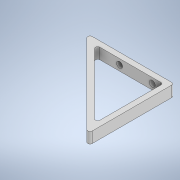
# Autodesk Inventor part: 25degbracketlcd
Saved by Autodesk Inventor 2020.2 (Build 242310000, 310)
## iProperties
Created: 2020-08-26
Part Number: 25degbracketlcd
Material: Generic
Document SubType Name: Modeling
Designer: JK
Density: 1 g/cm^3
Appearance: Default
Author: JK
Autodesk Inventor part; units mm, degrees
ref_plane "YZ Plane" through (0, 0, 0) normal (1, 0, 0) x (0, 1, 0)
ref_plane "XZ Plane" through (0, 0, 0) normal (0, 1, 0) x (-1, 0, 0)
ref_plane "XY Plane" through (0, 0, 0) normal (0, 0, 1) x (1, 0, 0)
sketch "Sketch1" plane through (0, 0, 0) normal (0, 1, 0) x (-1, 0, 0)
  line L0 (62.585, -18.917) -> (-13.8794, 57.5475)
  line L1 (-13.8794, 57.5475) -> (-13.8794, -22.4525)
  line L2 (-13.8794, -22.4525) -> (-8.8794, -22.4525)
  line L3 (-8.8794, -22.4525) -> (-8.8794, 45.4764)
  line L4 (-8.8794, 45.4764) -> (59.0495, -22.4525)
  line L5 (59.0495, -22.4525) -> (62.585, -18.917)
  line L6 (59.0495, -22.4525) -> (-8.8794, -22.4525)
  line L7 (-8.8794, -17.4525) -> (61.1206, -17.4525)
  line L8 (59.0495, -22.4525) -> (66.1206, -22.4525)
  line L9 (66.1206, -22.4525) -> (62.585, -18.917)
  point P0 (0, 0)
  point P1 (54.0495, -17.4525)
  dimension "d0" = 45
  dimension "d1" = 5
  dimension "d3" = 5
  dimension "d7" = 5
  dimension "d27" = 80
  constraints: 20 end point, 2 horizontal, 2 perpendicular, 2 point on line, 2 vertical, 1 collinear, 1 horizontal alignment, 1 parallel
  measures "d0" angle of L4 L3
  measures "d1" distance between parallel lines of L3 L1
  measures "d3" distance between parallel lines of L4 L0
  measures "d7" distance between parallel lines of L6 L7
  measures "d27" distance of L1.end L8.end
extrude "Extrusion1" add sketch "Sketch1" along normal blind 10 contours L5 L4 L7 L0 | L9 L8 L5 | L7 L4 L3 L2 L1 L0 | L6 L3 L7 L4
sketch "Sketch3" plane through (-54.0495, 0, -17.4525) normal (0, 0, 1) x (1, 0, 0)
  circle A0 centre (52.9289, 5) radius 2.75
  line L0 (0, 10) -> (62.9289, 10) projected
  line L1 (67.9289, 0) -> (67.9289, 10) projected
  circle A1 centre (22.9289, 5) radius 2.75
  point P0 (54.0495, 0)
  dimension "d16" = 5.5
  dimension "d17" = 5
  dimension "d18" = 15
  dimension "d22" = 30
  constraints: 2 centre point, 1 equal radius, 1 horizontal alignment
  measures "d16" diameter of A0
  measures "d17" distance from line of L0 A0.centre
  measures "d18" distance from line of A0.centre L1
  measures "d22" distance of A1.centre A0.centre
extrude "Extrusion3" cut sketch "Sketch3" against normal blind 10
sketch "Sketch5" plane through (13.8794, 0, 57.5475) normal (-0.7071068, 0, 0.7071068) x (0.7071068, 0, 0.7071068)
  circle A0 centre (-23, 5) radius 1.75
  circle A1 centre (-88, 5) radius 1.75
  line L0 (-113.1371, 10) -> (0, 10) projected
  line L1 (0, 0) -> (0, 10) projected
  point P0 (-50.5065, 0)
  dimension "d28" = 3.5
  dimension "d29" = 65
  dimension "d30" = 5
  dimension "d31" = 23
  constraints: 2 centre point, 1 equal radius, 1 horizontal alignment
  measures "d28" diameter of A1
  measures "d29" distance of A1.centre A0.centre
  measures "d30" distance from line of L0 A0.centre
  measures "d31" distance from line of L1 A0.centre
extrude "Extrusion5" cut sketch "Sketch5" against normal blind 10
fillet "Fillet2" radius 2 6 edges at (-66.1206, 5, -22.4525) (-54.0495, 5, -17.4525) (13.8794, 5, -22.4525) (13.8794, 5, 57.5475) (8.8794, 5, -17.4525) (8.8794, 5, 45.4764)
sketch "Sketch6" plane through (5.4652, 0, 42.0622) normal (0.7071068, 0, -0.7071068) x (-0.7071068, 0, -0.7071068)
  circle A0 centre (71.1005, 5) radius 1.75 projected
  circle A1 centre (71.1005, 5) radius 3
  circle A2 centre (6.1005, 5) radius 1.75 projected
  circle A3 centre (6.1005, 5) radius 3
  line L0 (74.5643, 5.0461) -> (72.8724, 2.0233)
  line L1 (72.8724, 2.0233) -> (69.4086, 1.9772)
  line L2 (69.4086, 1.9772) -> (67.6367, 4.9539)
  line L3 (67.6367, 4.9539) -> (69.3286, 7.9767)
  line L4 (69.3286, 7.9767) -> (72.7924, 8.0228)
  line L5 (72.7924, 8.0228) -> (74.5643, 5.0461)
  line L6 (9.5639, 5.0704) -> (7.8931, 2.0358)
  line L7 (7.8931, 2.0358) -> (4.4298, 1.9654)
  line L8 (4.4298, 1.9654) -> (2.6371, 4.9296)
  line L9 (2.6371, 4.9296) -> (4.3079, 7.9642)
  line L10 (4.3079, 7.9642) -> (7.7713, 8.0346)
  line L11 (7.7713, 8.0346) -> (9.5639, 5.0704)
  point P0 (33.607, 0)
  dimension "d35" = 6
  dimension "d36" = 6
  constraints: 24 end point, 4 coincident, 2 centre point, 2 tangent, 26 other
  measures "d35" diameter of A1
  measures "d36" diameter of A3
extrude "Extrusion6" cut sketch "Sketch6" against normal blind 2.5 contours A0 | A1 | A1 L5 L0 | A1 L4 L5 | L0 L1 A1 | A1 L3 L4 | L1 L2 A1 | A1 L2 L3 | A2 | A3 | A3 L11 L6 | A3 L10 L11 | L6 L7 A3 | A3 L9 L10 | L7 L8 A3 | A3 L8 L9
body "Solid1"
